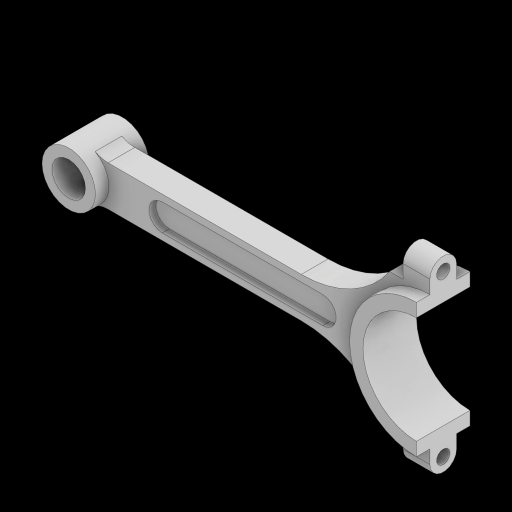
# Autodesk Inventor part: ANS7-3-BK
Saved by Autodesk Inventor 2024 (Build 280153000, 153)
## iProperties
Created: 2023-10-22
Part Number: ANS7-3-BK
Material: Generic
Document SubType Name: Modeling
Designer: bennk
Density: 1 g/cm^3
Appearance: Default
Mass: 53.1418 g
Surface Area: 207.395 cm^2
Volume: 53.1418 cm^3
Author: bennk
Autodesk Inventor part; units mm, degrees
ref_plane "YZ Plane" through (0, 0, 0) normal (1, 0, 0) x (0, 1, 0)
ref_plane "XZ Plane" through (0, 0, 0) normal (0, 1, 0) x (-1, 0, 0)
ref_plane "XY Plane" through (0, 0, 0) normal (0, 0, 1) x (1, 0, 0)
sketch "Sketch1" plane through (0, 0, 0) normal (0, 0, 1) x (1, 0, 0)
  arc A0 (0, 25.4) -> (0, -25.4) centre (0, 0) ccw
  circle A1 centre (-165.1, 0) radius 12.7
  line L0 (-165.1, 0) -> (0, 0) construction
  circle A2 centre (-165.1, 0) radius 7.9375
  arc A3 (0, 31.75) -> (0, -31.75) centre (0, 0) ccw
  line L1 (-156.6997, 9.525) -> (-61.0513, 9.525)
  line L2 (-156.6997, -9.525) -> (-30.2876, -9.525)
  line L3 (0, 25.4) -> (0, 44.45)
  line L4 (0, 44.45) -> (-12.7, 44.45)
  line L5 (-12.7, 44.45) -> (-12.7, 31.75)
  line L6 (-12.7, 31.75) -> (-19.05, 31.75)
  arc A4 (-61.0513, 9.525) -> (-19.05, 31.75) centre (-61.0513, 60.325) ccw
  line L7 (0, -25.4) -> (0, -44.45)
  line L8 (0, -44.45) -> (-12.7, -44.45)
  line L9 (-12.7, -44.45) -> (-12.7, -31.75)
  line L10 (-12.7, -31.75) -> (-19.05, -31.75)
  arc A5 (-19.05, -31.75) -> (-61.0513, -9.525) centre (-61.0513, -60.325) ccw
  point P0 (-6.35, 44.45)
  point P1 (-15.875, 31.75)
  point P2 (-61.0513, -9.525)
  dimension "d0" = 50.8
  dimension "d1" = 25.4
  dimension "d2" = 165.1
  dimension "d3" = 15.875
  dimension "d4" = 63.5
  dimension "d5" = 19.05
  dimension "d6" = 9.525
  dimension "d7" = 44.45
  dimension "d8" = 12.7
  dimension "d10" = 19.05
  dimension "d11" = 31.75
  dimension "d12" = 101.6
  constraints: 22 end point, 11 point on circle, 7 symmetric about line, 6 centre point, 3 coincident, 3 perpendicular, 3 point on line, 2 horizontal, 2 midpoint, 2 parallel, 1 tangent, 1 other
  measures "d0" diameter of A0
  measures "d1" diameter of A1
  measures "d2" distance of point (0, 0) L0.start
  measures "d3" diameter of A2
  measures "d4" diameter of A3
  measures "d5" distance between parallel lines of L1 L2
  measures "d6" distance between parallel lines of L0 L2
  measures "d7" distance from line of L0 point (-6.35, 44.45)
  measures "d8" distance between parallel lines of L5 L3
  measures "d10" distance from line of L3 L6.end
  measures "d11" vertical distance of point (0, 0) point (-15.875, 31.75)
  measures "d12" diameter of A4
extrude "CENTER WEB" add sketch "Sketch1" along normal mid plane 12.7 contours A3 L2 A1 L1 A4 L6 L5 L4 L3 | L7 L8 L9 L10 A5 L2 A3
extrude "END RINGS" add sketch "Sketch1" along normal mid plane 25.4 contours A0 L7 A3 L3 | A1
fillet "Fillet1" radius 12.7 2 edges at (-156.6997, 9.525, 0) (-156.6997, -9.525, 0)
fillet "Fillet2" radius 6.35 4 edges at (-6.35, 44.45, 6.35) (-6.35, 44.45, -6.35) (-6.35, -44.45, 6.35) (-6.35, -44.45, -6.35)
sketch "Sketch2" plane through (0, 25.4, 12.7) normal (1, 0, 0) x (0, 0, -1)
  arc A0 (19.05, 12.7) -> (6.35, 12.7) centre (12.7, 12.7) ccw projected
  point P0 (12.7, -25.4)
  constraints: 1 coincident
hole "Hole1" at (0, 38.1, 0) direction (-1, 0, 0) diameter 6.35 end through all
mirror "Mirror1" about plane through (0, 0, 0) normal (0, 1, 0) of "Hole1"
sketch "Sketch3" plane through (0, 0, 6.35) normal (0, 0, 1) x (1, 0, 0)
  line L0 (-127, 0) -> (-50.8, 0) construction
  line L1 (-61.0513, -9.525) -> (-152.8033, -9.525) projected
  line L2 (-127, 6.35) -> (-50.8, 6.35)
  line L3 (-50.8, -6.35) -> (-127, -6.35)
  arc A0 (-127, 6.35) -> (-127, -6.35) centre (-127, 0) ccw
  arc A1 (-50.8, -6.35) -> (-50.8, 6.35) centre (-50.8, 0) ccw
  point P0 (0, 0)
  point P1 (-88.9, 0)
  dimension "d27" = 6.35
  dimension "d28" = 76.2
  dimension "d29" = 50.8
  dimension "d30" = 6.35
  constraints: 8 end point, 4 point on circle, 4 tangent, 2 centre point, 2 parallel, 1 midpoint
  measures "d27" radius of A0
  measures "d28" distance of L0.start L0.end
  measures "d29" distance of point (0, 0) L0.end
  measures "d30" distance from line of point (0, 0) L2
extrude "RIGHT POCKET" cut sketch "Sketch3" against normal blind 3.175
mirror "Mirror2" about plane through (0, 0, 0) normal (0, 0, 1) of "RIGHT POCKET"
equation "\"d6\" = 0.5 * d5"
body "Solid1"
